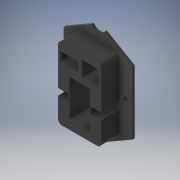
# Autodesk Inventor part: BA27
Saved by Autodesk Inventor 2017 (Build 210142000, 142)
## iProperties
Created: 2019-04-01
Part Number: BA27
Material: ABS Plastic
Document SubType Name: Modeling
Designer: Dell
Density: 1.06 g/cm^3
Appearance: Smooth - Black
Author: Dell
Autodesk Inventor part; units mm, degrees
ref_plane "YZ Plane" through (0, 0, 0) normal (1, 0, 0) x (0, 1, 0)
ref_plane "XZ Plane" through (0, 0, 0) normal (0, 1, 0) x (-1, 0, 0)
ref_plane "XY Plane" through (0, 0, 0) normal (0, 0, 1) x (1, 0, 0)
sketch "Sketch1" plane through (0, 0, 0) normal (0, 0, 1) x (1, 0, 0)
  line L0 (0, 0) -> (58, 0)
  line L1 (58, 0) -> (58, 98)
  line L2 (58, 98) -> (0, 98)
  line L3 (0, 98) -> (0, 0)
  line L4 (15, 62) -> (43, 62)
  line L5 (43, 62) -> (43, 12)
  line L6 (43, 12) -> (15, 12)
  line L7 (15, 12) -> (15, 62)
  circle A0 centre (9, 37) radius 2.5
  circle A1 centre (49, 37) radius 2.5
  line L8 (9, 37) -> (49, 37) construction
  line L9 (3, 86) -> (27, 86)
  line L10 (27, 86) -> (27, 74)
  line L11 (27, 74) -> (3, 74)
  line L12 (3, 74) -> (3, 86)
  circle A2 centre (-8.5, 49) radius 2.5
  circle A3 centre (66.5, 49) radius 2.5
  line L13 (-8.5, 49) -> (66.5, 49) construction
  circle A4 centre (-8.5, 49) radius 5 construction
  circle A5 centre (66.5, 49) radius 5 construction
  line L14 (0, 0) -> (-13.3155, 47.6544)
  line L15 (0, 98) -> (-13.3155, 50.3456)
  line L16 (58, 98) -> (71.3155, 50.3456)
  line L17 (58, 0) -> (71.3155, 47.6544)
  arc A6 (-13.3155, 50.3456) -> (-13.3155, 47.6544) centre (-8.5, 49) ccw
  arc A7 (71.3155, 47.6544) -> (71.3155, 50.3456) centre (66.5, 49) ccw
  line L18 (32, 90.5) -> (55, 90.5)
  line L19 (55, 90.5) -> (55, 69.5)
  line L20 (55, 69.5) -> (32, 69.5)
  line L21 (32, 69.5) -> (32, 90.5)
  line L22 (3, 80) -> (55, 80) construction
  point P0 (29, 62)
  point P1 (29, 98)
  point P2 (29, 37)
  point P3 (15, 37)
  point P4 (29, 49)
  point P5 (0, 49)
  point P6 (29, 80)
  dimension "d0" = 58
  dimension "d1" = 98
  dimension "d2" = 28
  dimension "d3" = 50
  dimension "d4" = 12
  dimension "d5" = 5
  dimension "d6" = 5
  dimension "d7" = 40
  dimension "d9" = 24
  dimension "d10" = 12
  dimension "d12" = 12
  dimension "d13" = 5
  dimension "d14" = 5
  dimension "d15" = 75
  dimension "d16" = 10
  dimension "d17" = 10
  dimension "d18" = 23
  dimension "d19" = 21
  dimension "d20" = 5
  constraints: 46 end point, 9 midpoint, 8 centre point, 8 parallel, 8 point on circle, 6 horizontal, 5 perpendicular, 5 tangent, 4 vertical alignment, 2 coincident, 2 concentric, 2 horizontal alignment
  measures "d0" distance of L2.end L1.end
  measures "d1" distance of L1.end L0.end
  measures "d2" distance of L5.end L6.end
  measures "d3" distance of L4.end L5.end
  measures "d4" distance between parallel lines of L0 L6
  measures "d5" diameter of A0
  measures "d6" diameter of A1
  measures "d7" distance of L8.end L8.start
  measures "d9" distance of L10.end L11.end
  measures "d10" distance of L9.end L10.end
  measures "d12" distance between parallel lines of L4 L11
  measures "d13" diameter of A2
  measures "d14" diameter of A3
  measures "d15" distance of L13.start L13.end
  measures "d16" diameter of A4
  measures "d17" diameter of A5
  measures "d18" distance of L18.start L18.end
  measures "d19" distance of L18.end L19.end
  measures "d20" distance between parallel lines of L21 L10
extrude "Extrusion1" add sketch "Sketch1" against normal blind 3
extrude "Extrusion2" add sketch "Sketch1" along normal blind 25 contours L3 L2 L1 L0
fillet "Fillet1" radius 5 4 edges at (58, 98, 12.5) (58, 0, 12.5) (0, 0, 12.5) (0, 98, 12.5)
sketch "Sketch2" plane through (0, 0, 0) normal (0, 0, 1) x (1, 0, 0)
  circle A0 centre (49, 37) radius 2.5 projected
  circle A1 centre (9, 37) radius 2.5 projected
  line L0 (0, 5) -> (0, 93) projected
  line L1 (0, 32.5) -> (13.5, 32.5)
  line L2 (13.5, 32.5) -> (13.5, 41.5)
  line L3 (13.5, 41.5) -> (0, 41.5)
  line L4 (0, 41.5) -> (0, 32.5)
  line L5 (58, 5) -> (58, 93) projected
  line L6 (58, 32.5) -> (44.5, 32.5)
  line L7 (44.5, 32.5) -> (44.5, 41.5)
  line L8 (44.5, 41.5) -> (58, 41.5)
  line L9 (58, 41.5) -> (58, 32.5)
  line L10 (15, 62) -> (15, 12) projected
  line L11 (43, 12) -> (43, 62) projected
  point P0 (0, 0)
  point P1 (13.5, 37)
  point P2 (44.5, 37)
  dimension "d29" = 4.5
  dimension "d30" = 4.5
  dimension "d31" = 9
  constraints: 16 end point, 4 horizontal alignment, 4 parallel, 2 horizontal, 2 midpoint, 2 perpendicular, 2 point on line
  measures "d29" distance from line of L2 A1.centre
  measures "d30" distance from line of L7 A0.centre
  measures "d31" distance between parallel lines of L6 L8
extrude "Extrusion3" cut sketch "Sketch2" along normal through all
sketch "Sketch3" plane through (0, 0, -3) normal (0, 0, -1) x (-1, 0, 0)
  circle A0 centre (-29, -5) radius 2.5 construction
  circle A1 centre (-29, 103) radius 2.5 construction
  line L0 (0, 98) -> (-58, 98) projected
  line L1 (-58, 0) -> (0, 0) projected
  line L2 (-58, 98) -> (-29.6325, 105.4187)
  line L3 (0, 98) -> (-28.3675, 105.4187)
  line L4 (0, 0) -> (-28.3675, -7.4187)
  line L5 (-58, 0) -> (-29.6325, -7.4187)
  arc A2 (-29.6325, -7.4187) -> (-28.3675, -7.4187) centre (-29, -5) ccw
  arc A3 (-28.3675, 105.4187) -> (-29.6325, 105.4187) centre (-29, 103) ccw
  point P0 (-29, 98)
  dimension "d34" = 5
  dimension "d35" = 5
  dimension "d36" = 5
  dimension "d37" = 5
  constraints: 8 end point, 8 point on circle, 6 tangent, 4 centre point, 2 vertical alignment, 1 concentric, 1 midpoint
  measures "d34" diameter of A0
  measures "d35" diameter of A1
  measures "d36" distance from line of L0 A1.centre
  measures "d37" distance from line of A0.centre L1
extrude "Extrusion4" add sketch "Sketch3" against normal blind 3
fillet "Fillet2" radius 5 4 edges at (0, 98, -1.5) (58, 98, -1.5) (58, 0, -1.5) (0, 0, -1.5)
sketch "Sketch4" plane through (0, 0, -3) normal (0, 0, -1) x (-1, 0, 0)
  line L0 (-15, 62) -> (-15, 12) projected
  line L1 (-15, 12) -> (-43, 12) projected
  line L2 (-43, 12) -> (-43, 62) projected
  line L3 (-43, 62) -> (-15, 62) projected
  line L4 (-32, 90.5) -> (-32, 69.5) projected
  line L5 (-32, 69.5) -> (-55, 69.5) projected
  line L6 (-55, 69.5) -> (-55, 90.5) projected
  line L7 (-55, 90.5) -> (-32, 90.5) projected
  line L8 (-3, 86) -> (-3, 74) projected
  line L9 (-3, 74) -> (-27, 74) projected
  line L10 (-27, 74) -> (-27, 86) projected
  line L11 (-27, 86) -> (-3, 86) projected
  circle A0 centre (-49, 37) radius 2.5 projected
  circle A1 centre (-9, 37) radius 2.5 projected
  circle A2 centre (-66.5, 49) radius 2.5 projected
  circle A3 centre (8.5, 49) radius 2.5 projected
  arc A4 (-2.7778, -0.7265) -> (0.7727, 2.7653) centre (-4.0429, 4.1109) ccw projected
  line L12 (0.7727, 2.7653) -> (13.3155, 47.6544) projected
  arc A5 (13.3155, 47.6544) -> (13.3155, 50.3456) centre (8.5, 49) ccw projected
  line L13 (13.3155, 50.3456) -> (0.7727, 95.2347) projected
  arc A6 (0.7727, 95.2347) -> (-2.7778, 98.7265) centre (-4.0429, 93.8891) ccw projected
  line L14 (-28.3675, 105.4187) -> (-2.7778, 98.7265) projected
  arc A7 (-28.3675, 105.4187) -> (-29.6325, 105.4187) centre (-29, 103) ccw projected
  line L15 (-55.2222, 98.7265) -> (-29.6325, 105.4187) projected
  arc A8 (-55.2222, 98.7265) -> (-58.7727, 95.2347) centre (-53.9571, 93.8891) ccw projected
  line L16 (-58.7727, 95.2347) -> (-71.3155, 50.3456) projected
  arc A9 (-71.3155, 50.3456) -> (-71.3155, 47.6544) centre (-66.5, 49) ccw projected
  line L17 (-71.3155, 47.6544) -> (-58.7727, 2.7653) projected
  arc A10 (-58.7727, 2.7653) -> (-55.2222, -0.7265) centre (-53.9571, 4.1109) ccw projected
  line L18 (-55.2222, -0.7265) -> (-29.6325, -7.4187) projected
  arc A11 (-29.6325, -7.4187) -> (-28.3675, -7.4187) centre (-29, -5) ccw projected
  line L19 (-28.3675, -7.4187) -> (-2.7778, -0.7265) projected
  arc A12 (-27.3554, 109.2885) -> (-30.6446, 109.2885) centre (-29, 103) ccw
  line L20 (-27.3554, 109.2885) -> (-1.7658, 102.5963)
  arc A13 (4.6251, 96.3111) -> (-1.7658, 102.5963) centre (-4.0429, 93.8891) ccw
  line L21 (4.6251, 96.3111) -> (17.168, 51.422)
  arc A14 (17.168, 46.578) -> (17.168, 51.422) centre (8.5, 49) ccw
  line L22 (17.168, 46.578) -> (4.6251, 1.6889)
  arc A15 (-1.7658, -4.5963) -> (4.6251, 1.6889) centre (-4.0429, 4.1109) ccw
  line L23 (-1.7658, -4.5963) -> (-27.3554, -11.2885)
  arc A16 (-30.6446, -11.2885) -> (-27.3554, -11.2885) centre (-29, -5) ccw
  line L24 (-30.6446, -11.2885) -> (-56.2342, -4.5963)
  arc A17 (-62.6251, 1.6889) -> (-56.2342, -4.5963) centre (-53.9571, 4.1109) ccw
  line L25 (-62.6251, 1.6889) -> (-75.168, 46.578)
  arc A18 (-75.168, 51.422) -> (-75.168, 46.578) centre (-66.5, 49) ccw
  line L26 (-75.168, 51.422) -> (-62.6251, 96.3111)
  arc A19 (-56.2342, 102.5963) -> (-62.6251, 96.3111) centre (-53.9571, 93.8891) ccw
  line L27 (-56.2342, 102.5963) -> (-30.6446, 109.2885)
  point P0 (0, 0)
  dimension "d41" = 4
  constraints: 16 end point, 16 point on circle, 8 centre point, 15 other
  measures "d41" distance between parallel lines of L15 L27
extrude "Extrusion5" add sketch "Sketch4" against normal blind 3 contours L20 A13 L21 A14 L22 A15 L23 A16 L24 A17 L25 A18 L26 A19 L27 A12
sketch "Sketch6" plane through (0, 0, -3) normal (0, 0, -1) x (-1, 0, 0)
  line L0 (-29, 118.6904) -> (17.5, 91.8437) construction
  line L1 (17.5, 91.8437) -> (17.5, 38.1501) construction
  line L2 (17.5, 38.1501) -> (-29, 11.3033) construction
  line L3 (-29, 11.3033) -> (-75.5, 38.1501) construction
  line L4 (-75.5, 38.1501) -> (-75.5, 91.8437) construction
  line L5 (-75.5, 91.8437) -> (-29, 118.6904) construction
  line L6 (-29, -20.6904) -> (-75.5, 6.1563) construction
  line L7 (-75.5, 6.1563) -> (-75.5, 59.8499) construction
  line L8 (-75.5, 59.8499) -> (-29, 86.6967) construction
  line L9 (-29, 86.6967) -> (17.5, 59.8499) construction
  line L10 (17.5, 59.8499) -> (17.5, 6.1563) construction
  line L11 (17.5, 6.1563) -> (-29, -20.6904) construction
  line L12 (-15, 12) -> (-43, 12) construction
  arc A0 (-75.168, 51.422) -> (-75.168, 46.578) centre (-66.5, 49) ccw construction
  line L13 (-75.5, 59.8499) -> (-75.5, 38.1501) construction
  line L14 (17.5, 59.8499) -> (17.5, 38.1501) construction
  arc A1 (17.168, 46.578) -> (17.168, 51.422) centre (8.5, 49) ccw construction
  arc A2 (4.6251, 96.3111) -> (-1.7658, 102.5963) centre (-4.0429, 93.8891) ccw construction
  arc A3 (-1.7658, -4.5963) -> (4.6251, 1.6889) centre (-4.0429, 4.1109) ccw construction
  line L15 (-72.6977, 49) -> (-55.2357, 96.3111)
  line L16 (-55.2357, 96.3111) -> (0, 98)
  line L17 (0, 98) -> (14.2585, 49.0151)
  line L18 (14.2585, 49.0151) -> (2.9964, 0)
  line L19 (2.9964, 0) -> (-59.2966, 2.9606)
  line L20 (-59.2966, 2.9606) -> (-72.6977, 49)
  line L21 (-75.5, 91.8437) -> (-75.5, 6.1563)
  line L22 (-75.5, 6.1563) -> (-29, -20.6904)
  line L23 (-29, -20.6904) -> (17.5, 6.1563)
  line L24 (17.5, 91.8437) -> (17.5, 6.1563)
  line L25 (17.5, 91.8437) -> (-29, 118.6904)
  line L26 (-29, 118.6904) -> (-75.5, 91.8437)
  point P0 (0, 0)
  point P1 (-29, 64.9969)
  point P2 (-29, 33.0031)
  point P3 (-29, 12)
  constraints: 52 end point, 3 collinear, 3 parallel, 3 tangent, 3 vertical, 2 vertical alignment, 1 midpoint, 26 other
extrude "Extrusion7" add sketch "Sketch6" against normal blind 3
sketch "Sketch7" plane through (0, 0, -3) normal (0, 0, -1) x (-1, 0, 0)
  line L0 (-75.5, 91.8437) -> (-29, 118.6904) projected
  circle A0 centre (-29, 118.6904) radius 10
  point P0 (0, 0)
  dimension "d48" = 20
  constraints: 1 centre point
  measures "d48" diameter of A0
extrude "Extrusion8" cut sketch "Sketch7" against normal through all
body "Solid1"
